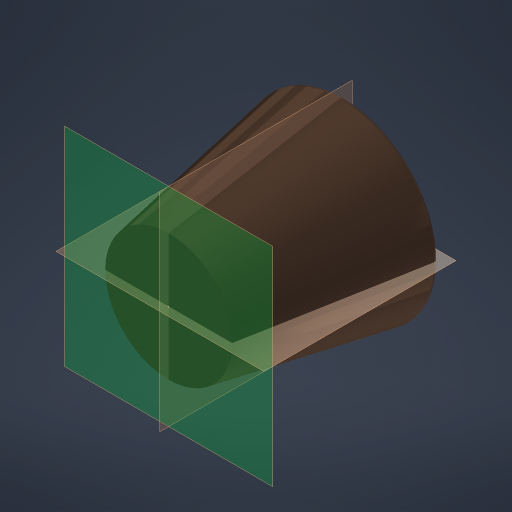
# Autodesk Inventor part: Flowerpot
Saved by Autodesk Inventor 2024 (Build 280153000, 153)
## iProperties
Manager: Louis Van Roosmaelen
Company: DCS - DIGITAL COMBAT SIMULATOR
Created: 2023-11-03
Part Number: Flowerpot
Material: S235
Catalog Web Link: http://emmausbovenbouw.op-weg.be/
Vendor: Emmaüsinstituut Bovenbouw Aalter
Document SubType Name: Modeling
Designer: Louis
Engineer: Declercq St.
Manufacturer: Standard
Standards Organization: Custom
Density: 7.86 g/cm^3
Appearance: Bronze - Satin
IDENT.NR.: AJ2022
TEAM: 30
Title: F18C Home Cockpit
Author: Louis
Keywords: Ø
Autodesk Inventor part; units mm, degrees
sketch "Sketch1" plane through (0, 0, 0) normal (0, 0, 1) x (1, 0, 0)
  line L0 (0, 2.8582) -> (0, -2.8582) construction
  line L1 (-5.7775, 0) -> (5.7775, 0) construction
  line L2 (0, 0) -> (-40, 0)
  line L3 (0, 0) -> (0, 110)
  line L4 (0, 110) -> (-60, 110)
  line L5 (-60, 110) -> (-40, 0)
  line L6 (-36, 4) -> (-55.2727, 110)
  line L7 (-36, 4) -> (0, 4)
  dimension "d0" = 40
  dimension "d1" = 110
  dimension "d2" = 60
  dimension "d3" = 36
  dimension "d4" = 4
  constraints: 16 end point, 3 point on line, 2 midpoint, 2 perpendicular, 2 vertical, 1 coincident, 1 horizontal, 1 parallel
  measures "d0" distance of L2.start L2.end
  measures "d1" distance of L2.start L3.end
  measures "d2" distance of L3.end L4.end
  measures "d3" distance of L6.start L7.end
  measures "d4" distance between parallel lines of L2 L7
revolve "Revolution1" add sketch "Sketch1" angle 360 about axis through (0, 0, 0) along (0, 1, 0) contours L2 L5 L4 L6 L7 L3
fillet "Fillet1" radius 2 1 edges at (60, 110, 0)
body "Solid1"
